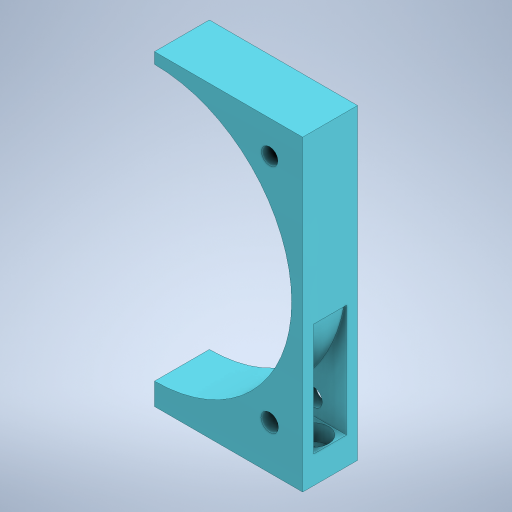
# Autodesk Inventor part: Aufnahme_Fan_02
Saved by Autodesk Inventor 2023.1 (Build 271208000, 208)
## iProperties
Created: 2023-12-09
Part Number: Aufnahme_Fan_02
Material: Generisch
Document SubType Name: Modeling
Designer: JansenL
Density: 1 g/cm^3
Appearance: Cadet Blue
Author: JansenL
Autodesk Inventor part; units mm, degrees
ref_plane "YZ Plane" through (0, 0, 0) normal (1, 0, 0) x (0, 1, 0)
ref_plane "XZ Plane" through (0, 0, 0) normal (0, 1, 0) x (-1, 0, 0)
sketch "Sketch1" plane through (0, 0, 0) normal (0, 0, 1) x (1, 0, 0)
  circle A0 centre (0, 0) radius 25 construction
  arc A1 (0, -25) -> (0, 25) centre (0, 0) ccw
  line L0 (0, 25) -> (0, 27)
  line L1 (0, 27) -> (27, 27)
  line L2 (27, 27) -> (27, -27)
  line L3 (27, -27) -> (0, -27)
  line L4 (0, -27) -> (0, -25)
  line L5 (0, 0) -> (27, 0) construction
  dimension "d0" = 50
  dimension "d2" = 27
  dimension "d4" = 54
  dimension "d5" = 2
  constraints: 12 end point, 5 perpendicular, 4 point on circle, 2 centre point, 2 coincident, 1 concentric, 1 midpoint, 1 point on line, 1 vertical, 1 other
  measures "d0" diameter of A0
  measures "d2" distance from line of L2 A0.centre
  measures "d4" distance between parallel lines of L3 L1
  measures "d5" distance of L0.start L0.end
extrude "Extrusion1" add sketch "Sketch1" along normal blind 10
ref_plane "Work Plane1" through (0, 0, 5) normal (0, 0, 1) x (1, 0, 0)
sketch "Sketch3" plane through (0, 0, 5) normal (0, 0, 1) x (1, 0, 0)
  line L0 (27, -27) -> (27, 27) projected
  line L1 (27, -24) -> (21, -24)
  line L2 (0, -27) -> (27, -27) projected
  line L3 (21, -24) -> (21, -16.5)
  line L4 (27, -4) -> (26.4915, -4)
  arc A0 (21, -16.5) -> (26.4915, -4) centre (-3, 1.5) ccw
  line L5 (27, -4) -> (27, -24)
  point P0 (0, 0)
  dimension "d17" = 3
  dimension "d18" = 20
  dimension "d19" = 30
  dimension "d20" = 1.5
  dimension "d21" = 3
  dimension "d22" = 6
  constraints: 8 end point, 2 point on circle, 2 point on line, 1 centre point, 1 collinear, 1 horizontal, 1 vertical
  measures "d17" distance between parallel lines of L2 L1
  measures "d18" distance between parallel lines of L1 L4
  measures "d19" radius of A0
  measures "d20" vertical distance of point (0, 0) A0.centre
  measures "d21" horizontal distance of point (0, 0) A0.centre
  measures "d22" distance between parallel lines of L0 L3
extrude "Extrusion3" cut sketch "Sketch3" along normal mid plane 6
sketch "Sketch4" plane through (0, 0, 10) normal (0, 0, 1) x (1, 0, 0)
  circle A0 centre (21, -21) radius 1.6
  point P0 (0, 0)
  dimension "d25" = 3.2
  dimension "d26" = 21
  dimension "d27" = 21
  constraints: 1 centre point
  measures "d25" diameter of A0
  measures "d26" horizontal distance of A0.centre point (0, 0)
  measures "d27" horizontal distance of A0.centre point (0, 0)
hole "Hole1" at (21, -21, 10) direction (0, 0, -1) diameter 3.2 depth 20 tip angle 118
chamfer "Chamfer2" distance 0.5 angle 45 1 edges at (27, -4, 5)
sketch "Sketch5" plane through (21, -24, 2) normal (0, 1, 0) x (1, 0, 0)
  circle A0 centre (3, -3) radius 1.6
  line L0 (11.4, -3) -> (-26.4, -3) projected
  line L1 (-21, 2) -> (-21, -8) projected
  circle A1 centre (3, -3) radius 2.75
  dimension "d38" = 3.2
  dimension "d39" = 24
  dimension "d40" = 5.5
  constraints: 2 centre point, 1 coincident, 1 point on line
  measures "d38" diameter of A0
  measures "d39" distance from line of L1 A0.centre
  measures "d40" diameter of A1
hole "Hole2" at (24, -24, 5) direction (0, -1, 0) diameter 3.2 depth 20 tip angle 118
extrude "Extrusion4" cut sketch "Sketch5" against normal blind 3 contours L0 A1 A0 | A0 L0 A1
sketch "Sketch6" plane through (0, 0, 10) normal (0, 0, 1) x (1, 0, 0)
  line L0 (0, -27) -> (27, -27)
  line L1 (27, -27) -> (27, -29)
  line L2 (27, -29) -> (0, -29)
  line L3 (0, -29) -> (0, -27)
  line L4 (27, -27) -> (27, 27) projected
  line L5 (0, -25) -> (0, -27) projected
  line L6 (0, -27) -> (27, -27) projected
  point P0 (0, 0)
  dimension "d50" = 2
  constraints: 8 end point, 3 collinear, 2 parallel, 1 horizontal, 1 perpendicular
  measures "d50" distance between parallel lines of L2 L0
extrude "Extrusion5" add sketch "Sketch6" against normal blind 10
hole "Hole3" at (24, -24, 5) direction (0, -1, 0) diameter 3.2 depth 20 tip angle 118
sketch "Sketch7" plane through (0, 0, 10) normal (0, 0, 1) x (1, 0, 0)
  line L0 (27, 27) -> (0, 27) projected
  line L1 (0, 27) -> (27, 27)
  line L2 (27, 27) -> (27, 24)
  line L3 (27, 24) -> (0, 24)
  line L4 (0, 24) -> (0, 27)
  line L5 (27, -29) -> (27, 27) projected
  point P0 (0, 0)
  dimension "d60" = 3
  constraints: 8 end point, 2 parallel, 1 collinear, 1 horizontal, 1 perpendicular
  measures "d60" distance between parallel lines of L3 L0
sketch "Sketch8" plane through (0, 0, 0) normal (0, 0, -1) x (-1, 0, 0)
  circle A0 centre (-21, 21) radius 1.85 projected
  circle A1 centre (-21, 21) radius 1.85 projected
  circle A2 centre (-21, 21) radius 1.85
  point P0 (0, 0)
  constraints: 1 centre point, 1 coincident, 1 concentric
hole "Hole4" at (21, 21, 0) direction (0, 0, 1) diameter 3 depth 10
body "Solid1"
